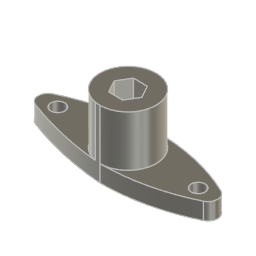
Practice problem 4 (Solidworks) (Autodesk Fusion 360 design; units mm, degrees)
Autodesk Fusion 360 part; units mm, degrees
sketch "Sketch1" plane through (0, 0, 0) normal (0, 0, 1) x (1, 0, 0)
  circle A0 centre (0, 0) radius 5.715
  line L0 (1.6335, 2.7225) -> (-1.541, 2.7759)
  line L1 (-1.541, 2.7759) -> (-3.1746, 0.0534)
  line L2 (-3.1746, 0.0534) -> (-1.6335, -2.7225)
  line L3 (-1.6335, -2.7225) -> (1.541, -2.7759)
  line L4 (1.541, -2.7759) -> (3.1746, -0.0534)
  line L5 (3.1746, -0.0534) -> (1.6335, 2.7225)
  circle A1 centre (0, 0) radius 6.35
  line L6 (0, 0) -> (-20.32, 0) construction
  line L7 (0, 0) -> (20.32, 0) construction
  line L8 (-20.32, 0) -> (-15.875, 0) construction
  line L9 (20.32, 0) -> (15.875, 0) construction
  circle A2 centre (15.875, 0) radius 1.5875
  circle A3 centre (-15.875, 0) radius 1.5875
  line L10 (-0.0017, -6.35) -> (-0.0017, 6.35) construction
  arc A4 (-0.0017, 6.35) -> (-19.0554, 2.0055) centre (0.0103, -37.6566) ccw
  arc A5 (-19.0554, -2.0055) -> (-0.0017, -6.35) centre (5.5821, 62.093) ccw
  arc A6 (-0.0017, -6.35) -> (19.0616, -2.0025) centre (0.0103, 37.5666) ccw
  arc A7 (19.0616, 2.0025) -> (-0.0017, 6.35) centre (0.0103, -37.5666) ccw
  arc A8 (19.0616, -2.0025) -> (19.0616, 2.0025) centre (18.0975, 0) ccw
  arc A9 (16.442, 1.4828) -> (15.875, 0) centre (18.0975, 0) ccw
  arc A10 (-19.0554, 2.0055) -> (-18.7183, -2.134) centre (-18.0975, 0) ccw
  dimension "d1" = 11.43
  dimension "d2" = 3.175
  dimension "d3" = 12.7
  dimension "d4" = 20.32
  dimension "d5" = 20.32
  dimension "d6" = 4.445
  dimension "d7" = 4.445
  dimension "d8" = 3.175
  dimension "d9" = 3.175
  constraint coincident A0.centre A1.centre
  constraint horizontal L6
  constraint parallel L6 L7
  constraint parallel L6 L8
  constraint parallel L7 L9
  constraint coincident L9.end A2.centre
  constraint coincident L8.end A3.centre
  constraint coincident A1 L10.start
  constraint coincident A1 L10.end
  constraint perpendicular L7 L10
  constraint midpoint L9 A8.centre
  constraint coincident L7.end A8
  constraint midpoint L8 A10.centre
  constraint coincident L6.end A10
  constraint tangent A1 A4
  constraint coincident A5.start A10
  constraint tangent A1 A6
  constraint tangent A6 A8
  constraint tangent A7 A8
  constraint tangent A1 A7
  constraint coincident A2 A9.start
  constraint concentric A8 A9
  constraint coincident A5 A10.end
  measures "d1" diameter of A0
  measures "d2" distance of L0.start A0.centre
  measures "d3" diameter of A1
  measures "d4" distance of A0.centre L6.end
  measures "d5" distance of A0.centre L7.end
  measures "d6" distance of L6.end L8.end
  measures "d7" distance of L7.end L9.end
  measures "d8" diameter of A2
  measures "d9" diameter of A3
extrude "Extrude1" add sketch "Sketch1" against normal blind 3.81 contours A0 | L0 L1 L2 L3 L4 L5 | A1 A5 | A1 A6 A7 A8 | A1 A4 A5 A10 picked at (-0.4559, 6.1097)
extrude "Extrude2" add sketch "Sketch1" along normal blind 11.43 contours A0 | A1 A5 picked at (-0.4559, 6.1097)
move_body "Move1" bodies 1 to x (1, 0, 0) y (0, 1, 0) z (0, 0, 1) at (0, 0, -11.43)
